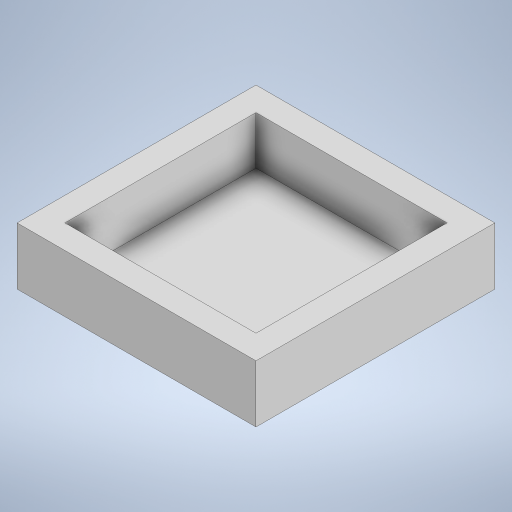
# Autodesk Inventor part: Box
Saved by Autodesk Inventor 2024.3 (Build 283343000, 343)
## iProperties
Created: 2025-06-26
Part Number: Box
Material: Generic
Document SubType Name: Modeling
Designer: 1
Density: 1 g/cm^3
Appearance: Default
Author: 1
Autodesk Inventor part; units mm, degrees
ref_plane "YZ Plane" through (0, 0, 0) normal (1, 0, 0) x (0, 1, 0)
ref_plane "XZ Plane" through (0, 0, 0) normal (0, 1, 0) x (-1, 0, 0)
ref_plane "XY Plane" through (0, 0, 0) normal (0, 0, 1) x (1, 0, 0)
sketch "Sketch1" plane through (0, 0, 0) normal (0, 1, 0) x (-1, 0, 0)
  line L0 (-125, 125) -> (125, 125)
  line L1 (125, 125) -> (125, -125)
  line L2 (125, -125) -> (-125, -125)
  line L3 (-125, -125) -> (-125, 125)
  line L4 (-125, 125) -> (125, -125) construction
  line L5 (125, 125) -> (-125, -125) construction
  point P0 (0, 0)
  dimension "d0" = 250
  constraints: 12 end point, 2 midpoint, 2 parallel, 2 perpendicular, 1 horizontal
  measures "d0" distance of L0.end L1.end
extrude "Extrusion1" add sketch "Sketch1" along normal mid plane 60
sketch "Sketch2" plane through (0, 30, 0) normal (0, 1, 0) x (1, 0, 0)
  line L0 (-100, -100) -> (100, -100)
  line L1 (100, -100) -> (100, 100)
  line L2 (100, 100) -> (-100, 100)
  line L3 (-100, 100) -> (-100, -100)
  line L4 (-100, -100) -> (100, 100) construction
  line L5 (100, -100) -> (-100, 100) construction
  point P0 (0, 0)
  dimension "d3" = 200
  constraints: 12 end point, 2 midpoint, 2 parallel, 2 perpendicular, 1 horizontal
  measures "d3" distance of L2.end L0.start
extrude "Extrusion2" cut sketch "Sketch2" against normal blind 50.4
body "Solid1"
